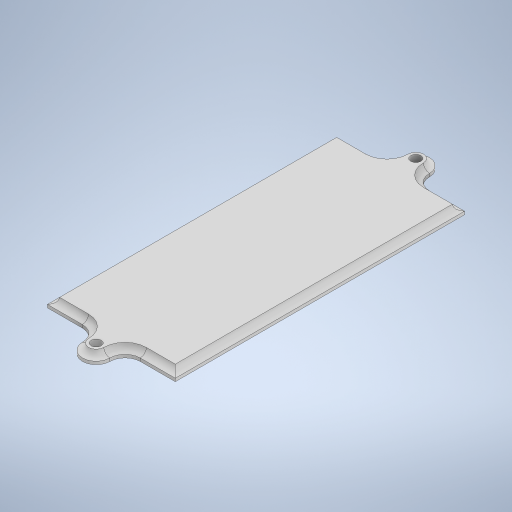
# Autodesk Inventor part: Cover
Saved by Autodesk Inventor 2024.2 (Build 282272000, 272)
## iProperties
Created: 2024-03-13
Part Number: Cover
Material: Generic
Document SubType Name: Modeling
Designer: jerem
Density: 1 g/cm^3
Appearance: Default
Author: jerem
Autodesk Inventor part; units mm, degrees
ref_plane "YZ Plane" through (0, 0, 0) normal (1, 0, 0) x (0, 1, 0)
ref_plane "XZ Plane" through (0, 0, 0) normal (0, 1, 0) x (-1, 0, 0)
ref_plane "XY Plane" through (0, 0, 0) normal (0, 0, 1) x (1, 0, 0)
sketch "Sketch1" plane through (0, 0, 0) normal (0, 1, 0) x (-1, 0, 0)
  line L0 (-21, -47.5) -> (21, -47.5)
  line L1 (21, -47.5) -> (21, 47.5)
  line L2 (21, 47.5) -> (-21, 47.5)
  line L3 (-21, 47.5) -> (-21, -47.5)
  line L4 (-21, -47.5) -> (21, 47.5) construction
  line L5 (21, -47.5) -> (-21, 47.5) construction
  circle A0 centre (0, 52.5) radius 1.65
  circle A1 centre (0, -52.5) radius 1.65
  circle A2 centre (0, 52.5) radius 4.5
  arc A3 (4.5, 52.5) -> (9.5, 47.5) centre (9.5, 52.5) ccw
  line L6 (0, 47.5) -> (0, 52.5) construction
  line L7 (21, 0) -> (-21, 0) construction
  arc A4 (9.5, -47.5) -> (4.5, -52.5) centre (9.5, -52.5) ccw
  line L8 (0, -47.5) -> (0, -52.5) construction
  circle A5 centre (0, -52.5) radius 4.5
  arc A6 (-9.5, 47.5) -> (-4.5, 52.5) centre (-9.5, 52.5) ccw
  arc A7 (-4.5, -52.5) -> (-9.5, -47.5) centre (-9.5, -52.5) ccw
  point P0 (0, 0)
  point P1 (-9.5, 47.5)
  point P2 (-9.5, -47.5)
  point P3 (-4.5, -52.5)
  point P4 (9.5, -47.5)
  dimension "d8" = 9
  dimension "d0" = 5
  dimension "d1" = 42
  dimension "d2" = 95
  dimension "d3" = 3.3
  dimension "d4" = 21
  dimension "d5" = 3.3
  dimension "d6" = 5
  dimension "d7" = 21
  dimension "d9" = 5
  constraints: 18 end point, 11 symmetric about line, 8 point on circle, 7 centre point, 5 midpoint, 2 parallel, 1 coincident, 1 horizontal, 1 perpendicular, 1 point on line, 1 tangent, 8 other
  measures "d0" distance of L6.start A0.centre
  measures "d1" distance of L1.end L2.end
  measures "d2" distance of L0.end L1.end
  measures "d3" diameter of A0
  measures "d4" horizontal distance of A0.centre L1.end
  measures "d5" diameter of A1
  measures "d6" distance from line of L0 A1.centre
  measures "d7" horizontal distance of L0.end A1.centre
  measures "d9" radius of A3
extrude "Extrusion1" add sketch "Sketch1" along normal blind 3
fillet "Fillet1" radius 2 12 edges at (21, 3, 0) (5.9645, 3, -48.9645) (0, 3, -57) (-5.9645, 3, -48.9645) (-15.25, 3, -47.5) (15.25, 3, -47.5) (-21, 3, 0) (0, 3, 57) (5.9645, 3, 48.9645) (15.25, 3, 47.5) (-15.25, 3, 47.5) (-5.9645, 3, 48.9645) inverted yes
equation "\"d5\" = d3"
equation "\"d6\" = d0"
body "Solid1"
